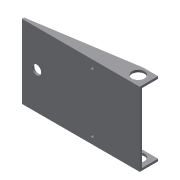
# Autodesk Inventor part: U-profil 100x40 - pod case
Saved by Autodesk Inventor 2015 (Build 190159000, 159)
## iProperties
Created: 2015-01-09
Part Number: U-profil 100x40 - pod case
Material: Všeobecné
Document SubType Name: Modeling
Designer: Michal
Density: 1 g/cm^3
Appearance: Výchozí
Author: Michal
Autodesk Inventor part; units mm, degrees
ref_plane "YZ Plane" through (0, 0, 0) normal (1, 0, 0) x (0, 1, 0)
ref_plane "XZ Plane" through (0, 0, 0) normal (0, 1, 0) x (-1, 0, 0)
ref_plane "XY Plane" through (0, 0, 0) normal (0, 0, 1) x (1, 0, 0)
sketch "Náčrt1" plane through (0, 0, 0) normal (1, 0, 0) x (0, 1, 0)
  line L0 (0, 0) -> (0, -100)
  line L1 (0, -100) -> (25, -100)
  line L2 (25, -100) -> (25, -97)
  line L3 (25, -97) -> (3, -97)
  line L4 (3, -97) -> (3, -3)
  line L5 (3, -3) -> (25, -3)
  line L6 (25, -3) -> (25, 0)
  line L7 (25, 0) -> (0, 0)
  dimension "d0" = 100
  dimension "d1" = 25
  dimension "d2" = 3
  dimension "d3" = 22
  dimension "d4" = 94
  dimension "d5" = 22
  dimension "d6" = 3
  constraints: 16 end point, 4 perpendicular, 2 point on line, 1 vertical
  measures "d0" distance of L0.start L0.end
  measures "d1" distance of L0.end L1.end
  measures "d2" distance of L1.end L2.end
  measures "d3" distance of L2.end L3.end
  measures "d4" distance of L3.end L4.end
  measures "d5" distance of L4.end L5.end
  measures "d6" distance of L5.end L6.end
extrude "Vysunutí1" add sketch "Náčrt1" along normal blind 160
sketch "Náčrt4" plane through (0, 3, -3) normal (0, 1, 0) x (1, 0, 0)
  line L0 (0, 94) -> (0, 0) projected
  line L1 (0, 0) -> (160, 0) projected
  line L2 (160, 94) -> (160, 0) projected
  line L3 (0, 94) -> (160, 94) projected
  circle A0 centre (20, 47) radius 6.25
  point P0 (0, -3)
  dimension "d30" = 12.5
  dimension "d31" = 47
  dimension "d32" = 20
  constraints: 1 centre point
  measures "d30" diameter of A0
  measures "d31" distance from line of L3 A0.centre
  measures "d32" distance from line of L0 A0.centre
extrude "Vysunutí4" cut sketch "Náčrt4" against normal through all contours A0
sketch "Náčrt6" plane through (0, 0, -100) normal (0, 0, -1) x (-1, 0, 0)
  circle A0 centre (-145, 13) radius 8.5
  line L0 (-160, 0) -> (-160, 25) projected
  line L1 (0, 25) -> (-160, 25) projected
  line L2 (0, 0) -> (-160, 0) projected
  dimension "d71" = 17
  dimension "d72" = 15
  dimension "d84" = 13
  constraints: 1 centre point
  measures "d71" diameter of A0
  measures "d72" distance from line of L0 A0.centre
  measures "d84" distance from line of A0.centre L2
extrude "Vysunutí6" cut sketch "Náčrt6" against normal through all
sketch "Náčrt7" plane through (0, 0, -100) normal (0, -1, 0) x (1, 0, 0)
  circle A0 centre (20, 50) radius 6.25 projected
  line L0 (0, 100) -> (0, 0) projected
  line L1 (0, 0) -> (160, 0) projected
  line L2 (160, 100) -> (160, 0) projected
  line L3 (0, 100) -> (160, 100) projected
  circle A1 centre (95, 90) radius 2.25
  circle A2 centre (95, 10) radius 2.25
  dimension "d76" = 4.5
  dimension "d77" = 4.5
  dimension "d78" = 10
  dimension "d79" = 10
  dimension "d80" = 95
  dimension "d81" = 95
  constraints: 2 centre point
  measures "d76" diameter of A1
  measures "d77" diameter of A2
  measures "d78" distance from line of L3 A1.centre
  measures "d79" distance from line of L1 A2.centre
  measures "d80" distance from line of A2.centre L0
  measures "d81" distance from line of L0 A1.centre
extrude "Vysunutí7" cut sketch "Náčrt7" against normal through all contours A1 | A2
sketch "Náčrt8" plane through (0, 0, -100) normal (0, 0, -1) x (-1, 0, 0)
  circle A0 centre (-145, 13) radius 8.5 projected
  line L0 (0, 0) -> (0, 25) projected
  line L1 (0, 25) -> (-160, 25) projected
  line L2 (-160, 0) -> (-160, 25) projected
  line L3 (0, 0) -> (-160, 0) projected
  line L4 (0, 3) -> (-160, 3) projected
  line L5 (0, 0) -> (0, 25) projected
  line L6 (0, 3) -> (-140, 25)
  line L7 (0, 25) -> (-160, 25) projected
  line L8 (0, 3) -> (0, 25)
  line L9 (0, 25) -> (-140, 25)
  dimension "d85" = 140
  dimension "d86" = 22
  constraints: 6 end point, 2 point on line, 1 collinear, 1 vertical
  measures "d85" distance from line of L0 L6.end
  measures "d86" distance from line of L6.start L1
extrude "Vysunutí8" cut sketch "Náčrt8" against normal through all contours L6 L1 L0
